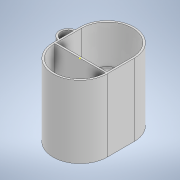
# Autodesk Inventor part: base-final
Saved by Autodesk Inventor 2021 (Build 250183000, 183)
## iProperties
Created: 2021-01-26
Part Number: base-final
Material: Generic
Document SubType Name: Modeling
Designer: Kayla
Density: 1 g/cm^3
Appearance: Default
Author: Kayla
Autodesk Inventor part; units mm, degrees
ref_plane "YZ Plane" through (0, 0, 0) normal (1, 0, 0) x (0, 1, 0)
ref_plane "XZ Plane" through (0, 0, 0) normal (0, 1, 0) x (-1, 0, 0)
ref_plane "XY Plane" through (0, 0, 0) normal (0, 0, 1) x (1, 0, 0)
sketch "Sketch1" plane through (0, 0, 0) normal (0, 1, 0) x (-1, 0, 0)
  line L0 (0, 0) -> (0, -60) construction
  line L1 (-60, 0) -> (-60, -60)
  line L2 (60, -60) -> (60, 0)
  arc A0 (60, 0) -> (-60, 0) centre (0, 0) ccw
  arc A1 (-60, -60) -> (60, -60) centre (0, -60) ccw
  point P0 (0, -30)
  dimension "d0" = 60
  dimension "d1" = 60
  constraints: 8 end point, 4 point on circle, 4 tangent, 2 centre point, 1 midpoint, 1 parallel, 1 vertical
  measures "d0" distance of L2.start L2.end
  measures "d1" radius of A1
extrude "Extrusion1" add sketch "Sketch1" along normal blind 160
sketch "Sketch2" plane through (0, 160, 0) normal (0, 1, 0) x (1, 0, 0)
  line L0 (0, 0) -> (0, 60) construction
  line L1 (56, 0) -> (56, 60)
  line L2 (-56, 60) -> (-56, 0)
  arc A0 (-56, 0) -> (56, 0) centre (0, 0) ccw
  arc A1 (56, 60) -> (-56, 60) centre (0, 60) ccw
  line L3 (-60, 60) -> (-60, 0) projected
  point P0 (0, 30)
  dimension "d5" = 4
  constraints: 8 end point, 4 point on circle, 4 tangent, 2 centre point, 1 midpoint, 1 parallel, 1 vertical
  measures "d5" distance between parallel lines of L3 L2
extrude "Extrusion2" cut sketch "Sketch2" against normal blind 86
sketch "Sketch3" plane through (0, 0, 0) normal (0, -1, 0) x (1, 0, 0)
  line L0 (0, 0) -> (0, -60) construction
  line L1 (-56, 0) -> (-56, -60)
  line L2 (56, -60) -> (56, 0)
  arc A0 (56, 0) -> (-56, 0) centre (0, 0) ccw
  arc A1 (-56, -60) -> (56, -60) centre (0, -60) ccw
  line L3 (60, 0) -> (60, -60) projected
  point P0 (0, -30)
  dimension "d8" = 4
  dimension "d9" = 60
  constraints: 8 end point, 4 point on circle, 4 tangent, 2 centre point, 1 midpoint, 1 parallel, 1 vertical
  measures "d8" distance between parallel lines of L3 L2
  measures "d9" distance of L2.start L2.end
extrude "Extrusion3" cut sketch "Sketch3" against normal blind 70
sketch "Sketch5" plane through (0, 160, 0) normal (0, 1, 0) x (1, 0, 0)
  arc A0 (-55.9943, 0) -> (55.9943, 0) centre (0, 0.0936) ccw
  line L0 (-55.9943, 0) -> (55.9943, 0)
  point P0 (0, 0)
  dimension "d14" = 111.9886
  constraints: 2 end point, 2 point on circle, 1 centre point, 1 horizontal
  measures "d14" distance of L0.end L0.start
extrude "Extrusion4" cut sketch "Sketch5" against normal blind 100
sketch "Sketch6" plane through (0, 74, 0) normal (0, 1, 0) x (1, 0, 0)
  line L0 (-56.7838, 0) -> (56.3732, 0)
  line L1 (56.3732, 0) -> (56.3732, 4)
  line L2 (56.3732, 4) -> (-56.7838, 4)
  line L3 (-56.7838, 4) -> (-56.7838, 0)
  point P0 (0, 0)
  dimension "d17" = 113.157
  dimension "d18" = 4
  constraints: 8 end point, 2 parallel, 1 horizontal, 1 perpendicular
  measures "d17" distance of L0.start L0.end
  measures "d18" distance of L2.end L0.start
extrude "Extrusion5" add sketch "Sketch6" along normal blind 86 and the other way blind 74
sketch "Sketch7" plane through (0, 0, 0) normal (0, -1, 0) x (1, 0, 0)
  arc A0 (57.3927, 0) -> (-56.9073, 0) centre (0.2427, -0.2605) ccw
  line L0 (57.3927, 0) -> (-56.9073, 0)
  point P0 (0, 0)
  dimension "d23" = 114.3
  constraints: 2 end point, 2 point on circle, 1 centre point, 1 horizontal
  measures "d23" distance of L0.end L0.start
extrude "Extrusion6" add sketch "Sketch7" against normal blind 4
sketch "Sketch8" plane through (0, 160, 0) normal (0, 1, 0) x (1, 0, 0)
  arc A0 (-56, 50) -> (-56, 10) centre (-56, 30) ccw
  line L0 (-56, 10) -> (-56, 50)
  arc A1 (60, 60) -> (-60, 60) centre (0, 60) ccw projected
  arc A2 (-60, 45.4919) -> (-60, 14.5081) centre (-56, 30) ccw
  line L1 (-60, 45.4919) -> (-60, 14.5081)
  line L2 (-56, 4) -> (-56, 60) projected
  point P0 (0, 0)
  dimension "d27" = 30
  dimension "d28" = 40
  dimension "d29" = 20
  dimension "d37" = 4
  dimension "d38" = 0
  constraints: 4 end point, 4 point on circle, 2 centre point, 1 vertical, 1 other
  measures "d27" vertical distance of A1.centre A0.centre
  measures "d28" distance of L0.start L0.end
  measures "d29" radius of A0
  measures "d37" distance between parallel lines of L0 L1
  measures "d38" distance between parallel lines of L2 L0
extrude "Extrusion7" add sketch "Sketch8" against normal blind 160
sketch "Sketch11" plane through (0, 0, 0) normal (0, -1, 0) x (1, 0, 0)
  line L0 (-60, -45.4919) -> (-56, -45.4919)
  line L1 (-56, -45.4919) -> (-56, -14.5081)
  line L2 (-56, -14.5081) -> (-60, -14.5081)
  line L3 (-60, -14.5081) -> (-60, -45.4919)
  line L4 (-60, -45.4919) -> (-60, -14.5081) projected
  point P0 (0, 0)
  dimension "d43" = 4
  dimension "d45" = 0
  dimension "d46" = 0
  dimension "d48" = 0
  constraints: 8 end point, 2 parallel, 1 horizontal, 1 perpendicular
  measures "d43" distance of L0.start L0.end
  measures "d45" distance between parallel lines of L4 L3
  measures "d46" distance from line of L0 L4.start
  measures "d48" distance from line of L2 L4.end
extrude "Extrusion8" cut sketch "Sketch11" against normal blind 50
sketch "Sketch12" plane through (0, 0, 0) normal (0, -1, 0) x (1, 0, 0)
  line L0 (-5, -4) -> (5, -4)
  line L1 (5, -4) -> (5, -14)
  line L2 (5, -14) -> (-5, -14)
  line L3 (-5, -14) -> (-5, -4)
  line L4 (-56, -4) -> (56, -4) projected
  line L5 (-5, -106) -> (5, -106)
  line L6 (5, -106) -> (5, -117)
  line L7 (5, -117) -> (-5, -117)
  line L8 (-5, -117) -> (-5, -106)
  arc A0 (-60, -60) -> (60, -60) centre (0, -60) ccw projected
  arc A1 (-56, -60) -> (56, -60) centre (0, -60) ccw
  point P0 (0, 0)
  point P1 (-5, -115.7763)
  point P2 (5, -115.7763)
  dimension "d51" = 10
  dimension "d52" = 10
  dimension "d53" = 0
  dimension "d54" = 5
  dimension "d55" = 11
  dimension "d56" = 10
  dimension "d57" = 5
  dimension "d58" = 3
  dimension "d63" = 56
  constraints: 16 end point, 4 parallel, 2 horizontal, 2 perpendicular, 2 point on circle, 1 centre point, 1 concentric
  measures "d51" distance of L2.end L0.start
  measures "d52" distance of L1.end L2.end
  measures "d53" distance between parallel lines of L4 L0
  measures "d54" distance from line of point (0, 0) L3
  measures "d55" distance of L7.end L5.start
  measures "d56" distance of L6.end L7.end
  measures "d57" distance from line of L8 point (0, 0)
  measures "d58" distance edge to line of A0 L7
  measures "d63" radius of A1
extrude "Extrusion11" add sketch "Sketch12" against normal blind 12.5 contours L0 L1 L2 L3 | L5 L6 A1 L8
extrude "Extrusion12" cut sketch "Sketch12" against normal blind 2 contours L0 L1 L2 L3 | L5 L6 A1 L8
sketch "Sketch16" plane through (0, 0, 0) normal (0, 0, 1) x (1, 0, 0)
  point P0 (0, 0)
sketch "Sketch17" plane through (0, 160, 0) normal (0, 1, 0) x (1, 0, 0)
  point P0 (0, 0)
body "Solid1"
